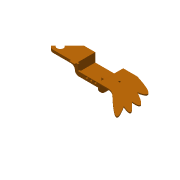
# Autodesk Inventor part: P_ankle02_001
Saved by Autodesk Inventor 2016 (Build 200138000, 138)
## iProperties
Created: 2016-02-23
Part Number: P_ankle02_001
Material: PC/ABS Plastic
Document SubType Name: Modeling
Designer: Mateusz
Density: 0.357273 g/cm^3
Appearance: Orange
Author: Mateusz
Autodesk Inventor part; units mm, degrees
ref_plane "YZ Plane" through (0, 0, 0) normal (1, 0, 0) x (0, 1, 0)
ref_plane "XZ Plane" through (0, 0, 0) normal (0, 1, 0) x (-1, 0, 0)
ref_plane "XY Plane" through (0, 0, 0) normal (0, 0, 1) x (1, 0, 0)
derived "skeleton.ipt"
sketch "Sketch1" plane through (0, 0, 0) normal (0, 0, 1) x (1, 0, 0)
  line L0 (9.8, -16) -> (3.2, -16) projected
  line L1 (3.2, 16) -> (9.8, 16) projected
  line L2 (38.5, 11.3) -> (38.5, 4.7) projected
  line L3 (38.5, -4.7) -> (38.5, -11.3) projected
  line L4 (-11.5, -0.1) -> (-11.5, -7) projected
  line L5 (-11.5, 7) -> (-11.5, 0.1) projected
  line L6 (-12.5, -0.1) -> (-12.5, -7)
  line L7 (39, -16.5) -> (-12.5, -16.5)
  line L8 (-12.5, -16.5) -> (-12.5, 16.5)
  line L9 (-12.5, 16.5) -> (39, 16.5)
  line L10 (39, 16.5) -> (39, -16.5)
  line L11 (-15, -19) -> (41.5, -19)
  line L12 (41.5, -19) -> (41.5, 19)
  line L13 (41.5, 19) -> (-15, 19)
  line L14 (-15, 19) -> (-15, -19)
  line L15 (-12.5, 0) -> (-15, 0)
  line L16 (39, 0) -> (41.5, -0.1)
  point P0 (0, 0)
  dimension "d0" = 1
  dimension "d1" = 0.5
  dimension "d2" = 0.5
  dimension "d3" = 0.5
  dimension "d4" = 2.5
  constraints: 22 end point, 5 parallel, 3 midpoint, 2 perpendicular, 1 collinear, 1 horizontal, 1 point on line, 3 other
  measures "d0" distance between parallel lines of L4 L6
  measures "d1" distance between parallel lines of L7 L0
  measures "d2" distance between parallel lines of L1 L9
  measures "d3" distance between parallel lines of L3 L10
  measures "d4" distance between parallel lines of L7 L11
extrude "Extrusion1" add sketch "Sketch1" along normal blind 32 contours L6 L8 L7 L10 L16 L12 L11 L14 L15
sketch "Sketch3" plane through (0, 0, 32) normal (0, 0, 1) x (1, 0, 0)
  line L0 (12.1, -10) -> (18.65, -10) projected
  line L1 (31.7, -10) -> (26.1, -10) projected
  line L2 (32.5, -4.8) -> (32.5, -9.2) projected
  line L3 (-15, -19) -> (41.5, -19) projected
  line L4 (41.5, -19) -> (41.5, -0.1) projected
  line L5 (-15, 0) -> (-15, -19) projected
  line L6 (-12.5, 0) -> (-15, 0) projected
  line L7 (-12.5, 0) -> (-15, 0) projected
  line L8 (-15, 0) -> (-15, -19) projected
  line L9 (-15, -19) -> (41.5, -19) projected
  line L10 (41.5, -19) -> (41.5, -0.1) projected
  line L11 (41.5, -0.1) -> (39, 0) projected
  line L12 (39, 0) -> (39, -16.5) projected
  line L13 (39, -16.5) -> (-12.5, -16.5) projected
  line L14 (-12.5, -16.5) -> (-12.5, 0) projected
  line L15 (39, 0) -> (39, -16.5) projected
  line L16 (-9.5, -11) -> (33.5, -11)
  line L17 (33.5, -11) -> (33.5, 0.22)
  line L18 (33.5, 0.22) -> (39, 0)
  line L19 (-12.5, 0) -> (-9.5, 0)
  line L20 (-9.5, 0) -> (-9.5, -11)
  line L21 (39, -16.5) -> (-12.5, -16.5) projected
  line L22 (-12.5, -16.5) -> (-12.5, 0) projected
  line L23 (41.5, -0.1) -> (39, 0) projected
  point P0 (0, 0)
  dimension "d7" = 1
  dimension "d8" = 1
  dimension "d9" = 1
  dimension "d10" = 3
  constraints: 11 end point, 3 parallel, 2 collinear, 2 perpendicular, 1 point on line
  measures "d7" distance between parallel lines of L0 L16
  measures "d8" distance between parallel lines of L16 L1
  measures "d9" distance between parallel lines of L17 L2
  measures "d10" distance between parallel lines of L14 L20
extrude "Extrusion2" add sketch "Sketch3" along normal blind 3
sketch "Sketch4" plane through (0, 0, 0) normal (0, 1, 0) x (-1, 0, 0)
  line L0 (-41.5, 0) -> (-41.5, 35) projected
  line L1 (15, 0) -> (15, 35) projected
  line L2 (58.316, 0) -> (-78.031, 0) projected
  line L3 (15, 35) -> (-41.5, 35) projected
  line L4 (0, -6.8) -> (0, 40.8) projected
  line L5 (15, 0) -> (15, 35) projected
  line L6 (15, 35) -> (60, 35)
  line L7 (60, 35) -> (60, 0)
  line L8 (60, 0) -> (15, 0)
  line L9 (15, 0) -> (15, 35)
  line L10 (-41.5, 35) -> (-60, 35)
  line L11 (-60, 35) -> (-60, 0)
  line L12 (-60, 0) -> (-41.5, 0)
  line L13 (-41.5, 0) -> (-41.5, 35)
  point P0 (0, 0)
  dimension "d17" = 120
  constraints: 16 end point, 4 parallel, 2 horizontal, 2 perpendicular, 2 point on line, 1 other
  measures "d17" distance between parallel lines of L11 L7
extrude "Extrusion3" add sketch "Sketch4" against normal blind 5 contours L2 L11 L10 L0 | L1 L6 L7 L8 L2
sketch "Sketch5" plane through (0, 0, 0) normal (0, 1, 0) x (-1, 0, 0)
  line L0 (0, -6.8) -> (0, 40.8) projected
  line L1 (93.2488, 0) -> (-139.4925, 0)
  point P0 (0, 0)
  point P1 (49, 23)
  dimension "d18" = 23
  dimension "d19" = 49
  constraints: 2 end point, 1 horizontal, 2 other
  measures "d18" distance from line of L1 point (49, 23)
  measures "d19" distance from line of point (49, 23) L0
hole "Hole1" at (-49, 0, 23) direction (0, -1, 0) diameter 12 end through all
sketch "Sketch6" plane through (0, 0, 35) normal (0, 0, 1) x (1, 0, 0)
  circle A0 centre (36, -8) radius 1.3 projected
  line L0 (2, 11.5) -> (-5.5, 11.5) projected
  arc A1 (-5.5, 11.5) -> (-10, 7) centre (-5.5, 7) ccw projected
  line L1 (-10, 7) -> (-10, -7) projected
  arc A2 (-10, -7) -> (-5.5, -11.5) centre (-5.5, -7) ccw projected
  line L2 (-5.5, -11.5) -> (2, -11.5) projected
  line L3 (2, -11.5) -> (2, -12.6) projected
  line L4 (2, -12.6) -> (3.2, -12.6) projected
  line L5 (3.2, -14.9) -> (3.2, -12.6) projected
  line L6 (3.2, -14.9) -> (9.8, -14.9) projected
  line L7 (9.8, -12.6) -> (9.8, -14.9) projected
  line L8 (9.8, -12.6) -> (11.2, -12.6) projected
  line L9 (11.2, -12.6) -> (11.2, -14.9) projected
  line L10 (11.2, -14.9) -> (17.8, -14.9) projected
  line L11 (17.8, -12.6) -> (17.8, -14.9) projected
  line L12 (17.8, -12.6) -> (19.2, -12.6) projected
  line L13 (19.2, -12.6) -> (19.2, -14.9) projected
  line L14 (19.2, -14.9) -> (25.8, -14.9) projected
  line L15 (25.8, -12.6) -> (25.8, -14.9) projected
  line L16 (25.8, -12.6) -> (27.2, -12.6) projected
  line L17 (27.2, -12.6) -> (27.2, -14.9) projected
  line L18 (27.2, -14.9) -> (33.8, -14.9) projected
  line L19 (33.8, -12.6) -> (33.8, -14.9) projected
  line L20 (33.8, -12.6) -> (35.0198, -12.6) projected
  arc A3 (35.0198, -12.6) -> (35.1, -12.5198) centre (34, -11.5) ccw projected
  line L21 (35.1, -12.5198) -> (35.1, -11.3) projected
  line L22 (35.1, -11.3) -> (37.4, -11.3) projected
  line L23 (37.4, -11.3) -> (37.4, -4.7) projected
  line L24 (35.1, -4.7) -> (37.4, -4.7) projected
  line L25 (35.1, 4.7) -> (35.1, -4.7) projected
  line L26 (35.1, 4.7) -> (37.4, 4.7) projected
  line L27 (37.4, 4.7) -> (37.4, 11.3) projected
  line L28 (35.1, 11.3) -> (37.4, 11.3) projected
  line L29 (35.1, 12.5198) -> (35.1, 11.3) projected
  arc A4 (35.1, 12.5198) -> (35.0198, 12.6) centre (34, 11.5) ccw projected
  line L30 (33.8, 12.6) -> (35.0198, 12.6) projected
  line L31 (33.8, 12.6) -> (33.8, 14.9) projected
  line L32 (33.8, 14.9) -> (27.2, 14.9) projected
  line L33 (27.2, 12.6) -> (27.2, 14.9) projected
  line L34 (25.8, 12.6) -> (27.2, 12.6) projected
  line L35 (25.8, 12.6) -> (25.8, 14.9) projected
  line L36 (25.8, 14.9) -> (19.2, 14.9) projected
  line L37 (19.2, 12.6) -> (19.2, 14.9) projected
  line L38 (17.8, 12.6) -> (19.2, 12.6) projected
  line L39 (17.8, 12.6) -> (17.8, 14.9) projected
  line L40 (17.8, 14.9) -> (11.2, 14.9) projected
  line L41 (11.2, 12.6) -> (11.2, 14.9) projected
  line L42 (9.8, 12.6) -> (11.2, 12.6) projected
  line L43 (9.8, 12.6) -> (9.8, 14.9) projected
  line L44 (9.8, 14.9) -> (3.2, 14.9) projected
  line L45 (3.2, 12.6) -> (3.2, 14.9) projected
  line L46 (2, 12.6) -> (3.2, 12.6) projected
  line L47 (2, 12.6) -> (2, 11.5) projected
  circle A5 centre (0, 0) radius 5.5 projected
  line L48 (12.1, -10) -> (18.65, -10) projected
  line L49 (12.1, -10) -> (12.1, 10) projected
  line L50 (18.65, 10) -> (12.1, 10) projected
  line L51 (18.65, -10) -> (18.65, 10) projected
  line L52 (26.1, -10) -> (31.7, -10) projected
  arc A6 (25.3, -9.2) -> (26.1, -10) centre (26.1, -9.2) ccw projected
  line L53 (25.3, -4.8) -> (25.3, -9.2) projected
  arc A7 (26.1, -4) -> (25.3, -4.8) centre (26.1, -4.8) ccw projected
  line L54 (31.7, -4) -> (26.1, -4) projected
  arc A8 (32.5, -4.8) -> (31.7, -4) centre (31.7, -4.8) ccw projected
  line L55 (32.5, -9.2) -> (32.5, -4.8) projected
  arc A9 (31.7, -10) -> (32.5, -9.2) centre (31.7, -9.2) ccw projected
  line L56 (31.7, 10) -> (26.1, 10) projected
  arc A10 (32.5, 9.2) -> (31.7, 10) centre (31.7, 9.2) ccw projected
  line L57 (32.5, 4.8) -> (32.5, 9.2) projected
  arc A11 (31.7, 4) -> (32.5, 4.8) centre (31.7, 4.8) ccw projected
  line L58 (26.1, 4) -> (31.7, 4) projected
  arc A12 (25.3, 4.8) -> (26.1, 4) centre (26.1, 4.8) ccw projected
  line L59 (25.3, 9.2) -> (25.3, 4.8) projected
  arc A13 (26.1, 10) -> (25.3, 9.2) centre (26.1, 9.2) ccw projected
  circle A14 centre (6.5, 13.5) radius 1.3 projected
  circle A15 centre (14.5, 13.5) radius 1.3 projected
  circle A16 centre (22.5, 13.5) radius 1.3 projected
  circle A17 centre (30.5, 13.5) radius 1.3 projected
  circle A18 centre (36, 8) radius 1.3 projected
  circle A19 centre (36, -8) radius 1.3 projected
  circle A20 centre (30.5, -13.5) radius 1.3 projected
  circle A21 centre (22.5, -13.5) radius 1.3 projected
  circle A22 centre (14.5, -13.5) radius 1.3 projected
  circle A23 centre (6.5, -13.5) radius 1.3 projected
  circle A24 centre (22, 8) radius 1.05 projected
  circle A25 centre (22, -8) radius 1.05 projected
  circle A26 centre (6, 8) radius 1.05 projected
  circle A27 centre (6, -8) radius 1.05 projected
  circle A28 centre (-7.7697, 6.2629) radius 1.05 projected
  circle A29 centre (-7.7697, -6.2629) radius 1.05 projected
  point P0 (0, 0)
  constraints: 5 coincident
hole "Hole2" at (6.5, -13.5, 35) at (14.5, -13.5, 35) at (22.5, -13.5, 35) at (30.5, -13.5, 35) at (36, -8, 35) direction (0, 0, -1) diameter 2.6 end through all
chamfer "Chamfer1" distance 1 angle 45 5 edges at (6.5, -12.2, 35) (14.5, -12.2, 35) (22.5, -12.2, 35) (30.5, -12.2, 35) (36, -6.7, 35)
sketch "Sketch8" plane through (0, 0, 0) normal (0, 1, 0) x (-1, 0, 0)
  line L0 (0, -22.074) -> (0, 132.4443) projected
  line L1 (104.6039, 0) -> (-172.6236, 0) projected
  point P0 (0, 0)
  point P1 (-52, 24.5788)
  dimension "d45" = 52
  measures "d45" distance from line of L0 point (-52, 24.579)
hole "Hole3" at (52, 0, 24.5788) direction (0, -1, 0) diameter 3.3 end through all
chamfer "Chamfer2" distance 1.5 angle 45 1 edges at (-49, -5, 17)
sketch "Sketch7" plane through (0, 0, 0) normal (0, 1, 0) x (-1, 0, 0)
  line L0 (-60, 0) -> (-60, 35) projected
  line L1 (84, 0) -> (-84, 0)
  line L2 (0, -10.7219) -> (0, 64.3314) projected
  spline S0 degree 2 poles (-60, 0) (-119.4007, 18.5193) (-85, 25) knots 0 0 0 1 1 1
  spline S1 degree 2 poles (-85, 25) (-126.077, 47.9796) (-95, 45) knots 0 0 0 1 1 1
  spline S2 degree 2 poles (-95, 45) (-126.5193, 73.2233) (-95, 60) knots 0 0 0 1 1 1
  spline S3 degree 2 poles (-95, 60) (-127.3392, 111.6615) (-60, 46) knots 0 0 0 1 1 1
  line L3 (-60, 35) -> (-60, 46)
  line L4 (-60, 35) -> (-41.5, 35) projected
  point P0 (0, 0)
  point P1 (-97.6161, 18.6161)
  point P2 (-108.3286, 43.1894)
  point P3 (-110.591, 63.5266)
  point P4 (-105.0007, 82.5034)
  dimension "d37" = 85
  dimension "d38" = 95
  dimension "d39" = 25
  dimension "d40" = 45
  dimension "d41" = 60
  dimension "d42" = 95
  dimension "d61" = 11
  constraints: 4 end point, 1 horizontal, 1 vertical, 14 other
  measures "d37" distance from line of point (-85, 25) L2
  measures "d38" distance from line of L2 point (-95, 45)
  measures "d39" distance from line of L1 point (-85, 25)
  measures "d40" distance from line of L1 point (-95, 45)
  measures "d41" distance from line of L1 point (-95, 60)
  measures "d42" distance from line of L2 point (-95, 60)
  measures "d61" distance of L0.end L3.end
extrude "Extrusion4" add sketch "Sketch7" against normal blind 2
sketch "Sketch9" plane through (0, 0, 35) normal (0, 0, 1) x (1, 0, 0)
  line L0 (60, -5) -> (41.5, -5) projected
  line L1 (41.5, -19) -> (41.5, -5) projected
  line L2 (-15, -19) -> (41.5, -19) projected
  line L3 (41.5, 0) -> (60, 0) projected
  line L4 (60, 0) -> (60, -2)
  line L5 (60, -2) -> (41.5, -2)
  line L6 (-15, -19) -> (41.5, -19) projected
  line L7 (41.5, -2) -> (41.5, -19)
  line L8 (41.5, -19) -> (38.5, -19)
  line L9 (60, 0) -> (41.5, 0) projected
  line L10 (38.5, 0) -> (60, 0)
  line L11 (38.5, -19) -> (38.5, 0)
  line L12 (41.5, -5) -> (60, -5) projected
  line L13 (60, -5) -> (60, 0)
  point P0 (0, 0)
  dimension "d56" = 3
  dimension "d60" = 2
  constraints: 14 end point, 3 perpendicular, 2 horizontal, 2 point on line
  measures "d56" distance between parallel lines of L1 L11
  measures "d60" distance between parallel lines of L3 L5
extrude "Extrusion5" add sketch "Sketch9" along normal blind 11 contours L1 L2 L11 L10 L3 L4 L5 L7
chamfer "Chamfer3" distance 3 angle 45 2 edges at (50.75, -5, 35) (60, -5, 17.5)
fillet "Fillet1" radius 20 1 edges at (60, -1, 46)
fillet "Fillet2" radius 10 1 edges at (40, -19, 46)
fillet "Fillet4" radius 10 1 edges at (-60, -2.5, 35)
fillet "Fillet7" radius 7 2 edges at (-15, -19, 17.5) (-15, -5, 17.5)
sketch "Sketch10" plane through (0, 0, 0) normal (0, 0, 1) x (1, 0, 0)
  line L0 (-15, -19) -> (38.5, -19) projected
  line L1 (-60, 0) -> (-60, -5) projected
  line L2 (-50, -5) -> (-60, -5) projected
  arc A0 (-15, -12) -> (-8, -19) centre (-8, -12) ccw projected
  line L3 (-9.8511, -18.7508) -> (-60, -5)
  line L4 (-22, -5) -> (-50, -5) projected
  arc A1 (-15, -12) -> (-22, -5) centre (-22, -12) ccw projected
  point P0 (0, 0)
  constraints: 2 end point, 1 point on circle, 1 tangent
extrude "Extrusion6" add sketch "Sketch10" along normal blind 3
sketch "Sketch11" plane through (0, 0, 3) normal (0, 0, 1) x (1, 0, 0)
  point P0 (0, 0)
  point P1 (-27.57, -9.8473)
hole "Hole4" at (-27.57, -9.8473, 3) direction (0, 0, -1) diameter 3.3 end through all
chamfer "Chamfer4" distance 1 angle 45 1 edges at (-27.57, -8.1973, 3)
fillet "Fillet9" radius 1 3 edges at (-17.0503, -7.0503, 3) (-13.5659, -16.2451, 3) (-41, -5, 3)
sketch "Sketch12" plane through (0, 0, 35) normal (0, 0, 1) x (1, 0, 0)
  circle A0 centre (36, -8) radius 2.3 projected
  circle A1 centre (22.5, -13.5) radius 2.3 projected
  circle A2 centre (6.5, -13.5) radius 2.3 projected
  arc A3 (-15, -12) -> (-8, -19) centre (-8, -12) ccw projected
  line L0 (-8, -19) -> (38.5, -19) projected
  line L1 (38.5, -19) -> (38.5, 0) projected
  line L2 (38.5, 0) -> (39, 0) projected
  line L3 (39, 0) -> (33.5, 0.22) projected
  line L4 (33.5, 0.22) -> (33.5, -11) projected
  line L5 (33.5, -11) -> (-9.5, -11) projected
  line L6 (-9.5, -11) -> (-9.5, 0) projected
  line L7 (-9.5, 0) -> (-50, 0) projected
  line L8 (-50, -5) -> (-50, 0) projected
  line L9 (-22, -5) -> (-50, -5) projected
  arc A4 (-15, -12) -> (-22, -5) centre (-22, -12) ccw projected
  circle A5 centre (14.5, -13.5) radius 2.3 projected
  circle A6 centre (30.5, -13.5) radius 2.3 projected
  line L10 (-12.5, -16.5) -> (-12.5, 0) projected
  line L11 (-12.5, 0) -> (-15.5, 0)
  line L12 (-15.5, 0) -> (-15.5, -5)
  line L13 (-15.5, -5) -> (-12.5, -5)
  line L14 (-12.5, -5) -> (-12.5, 0)
  point P0 (0, 0)
  dimension "d86" = 3
  dimension "d87" = 5
  constraints: 8 end point, 2 parallel, 1 horizontal, 1 perpendicular
  measures "d86" distance between parallel lines of L12 L14
  measures "d87" distance between parallel lines of L11 L13
extrude "Extrusion7" add sketch "Sketch12" along normal blind 3 contours L7 L10 L13 L12
equation "\"d19\" = ankle_length"
equation "\"ankle_length\" = 49"
body "Solid1"
